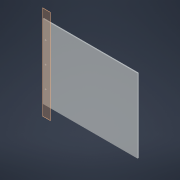
# Autodesk Inventor part: front-glass
Saved by Autodesk Inventor 2021 (Build 250183000, 183)
## iProperties
Created: 2020-05-11
Part Number: front-glass
Material: Glass
Document SubType Name: Modeling
Designer: Jonathan
Mass: 318.351 g
Surface Area: 1000.23 cm^2
Volume: 146.032 cm^3
Density: 2.18 g/cm^3
Appearance: Clear
Author: Jonathan
Autodesk Inventor part; units mm, degrees
ref_plane "YZ Plane" through (0, 0, 0) normal (1, 0, 0) x (0, 1, 0)
ref_plane "XZ Plane" through (0, 0, 0) normal (0, 1, 0) x (-1, 0, 0)
ref_plane "XY Plane" through (0, 0, 0) normal (0, 0, 1) x (1, 0, 0)
ref_plane "Work Plane1" through (0, 0, 0) normal (0, 0, 1) x (1, 0, 0)
sketch "Sketch1" plane through (0, 0, 0) normal (0, 0, 1) x (1, 0, 0)
  line L0 (3, 20) -> (253, 20)
  line L1 (253, 20) -> (253, 214.71)
  line L2 (253, 214.71) -> (3, 214.71)
  line L3 (3, 214.71) -> (3, 20)
  circle A0 centre (9.5, 56.25) radius 1.6 construction
  circle A1 centre (9.5, 112.5) radius 1.6 construction
  circle A2 centre (9.5, 168.75) radius 1.6 construction
  line L4 (19, 225) -> (19, 0) construction
  line L5 (19, 225) -> (13.5011, 225) construction
  ellipse E0 centre (12.5333, 224.7099) end of major axis (12.5333, 225.8617) minor radius 1 (13.5333, 224.7099) -> (13.5011, 225) ccw construction
  line L6 (13.5333, 219.5971) -> (13.5333, 224.7099) construction
  ellipse E1 centre (12.5333, 219.5971) end of major axis (12.5333, 217.71) minor radius 1 (12.5333, 217.71) -> (13.5333, 219.5971) ccw construction
  line L7 (7.4667, 217.71) -> (12.5333, 217.71) construction
  ellipse E2 centre (7.4667, 219.5971) end of major axis (7.4667, 217.71) minor radius 1 (6.4667, 219.5971) -> (7.4667, 217.71) ccw construction
  line L8 (6.4667, 224.7099) -> (6.4667, 219.5971) construction
  ellipse E3 centre (7.4667, 224.7099) end of major axis (7.4667, 225.8617) minor radius 1 (6.4989, 225) -> (6.4667, 224.7099) ccw construction
  line L9 (6.4989, 225) -> (0, 225) construction
  line L10 (0, 0) -> (0, 225) construction
  line L11 (0, 0) -> (19, 0) construction
  dimension "d0" = 3
  dimension "d1" = 3
  dimension "d2" = 250
  dimension "d3" = 20
  constraints: 8 end point, 2 parallel, 1 horizontal, 1 perpendicular, 4 other
  measures "d0" distance between parallel lines of L7 L2
  measures "d1" distance between parallel lines of L10 L3
  measures "d2" distance of L1.end L2.end
  measures "d3" distance between parallel lines of L11 L0
extrude "Extrusion1" add sketch "Sketch1" along normal blind 3
sketch "Sketch2" plane through (0, 0, 3) normal (0, 0, 1) x (1, 0, 0)
  circle A0 centre (9.5, 168.75) radius 1.6 projected
  circle A1 centre (9.5, 112.5) radius 1.6 projected
  circle A2 centre (9.5, 56.25) radius 1.6 projected
  point P0 (0, 0)
extrude "Extrusion2" cut sketch "Sketch2" against normal through all
equation "\"d1\" = d0"
body "Solid1"
